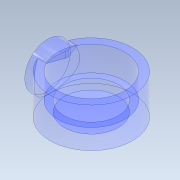
# Autodesk Inventor part: hip_right
Saved by Autodesk Inventor 2020 (Build 240168000, 168)
## iProperties
Created: 2021-03-27
Part Number: hip_right
Material: Generic
Document SubType Name: Modeling
Designer: DELL
Density: 1 g/cm^3
Appearance: Clear - Blue
Author: DELL
Autodesk Inventor part; units mm, degrees
ref_plane "YZ Plane" through (0, 0, 0) normal (1, 0, 0) x (0, 1, 0)
ref_plane "XY Plane" through (0, 0, 0) normal (0, 0, 1) x (1, 0, 0)
ref_plane "UCS1: YZ Plane" through (0, 0, 0) normal (1, 0, 0) x (0, 1, 0)
sketch "Sketch2" plane through (0, 0, 0) normal (1, 0, 0) x (0, 1, 0)
  circle A0 centre (0, 0) radius 26.5
  dimension "d0" = 53
  constraints: 1 centre point, 1 coincident
  measures "d0" diameter of A0
extrude "Extrusion1" add sketch "Sketch2" along normal blind 51
sketch "Sketch3" plane through (0, 0, 0) normal (0, 1, 0) x (-1, 0, 0)
  line L0 (-51, 26.5) -> (-51, -26.5) projected
  circle A0 centre (-51, 0) radius 48
  circle A1 centre (-51, 0) radius 39
  line L1 (-16.6387, 18.4473) -> (-22.6683, 1.8811)
  circle A2 centre (-17.5, 0) radius 5.5
  line L2 (0, 0) -> (-51, 0) construction
  line L3 (0, 26.5) -> (0, -26.5) construction
  line L4 (-16.6387, -18.4473) -> (-22.6683, -1.8811)
  circle A3 centre (-51, 0) radius 31.5
  point P0 (-22.6683, -1.8811)
  point P1 (-20.4946, 7.8532)
  point P2 (-20.4946, -7.8532)
  dimension "d4" = 78
  dimension "d7" = 11
  dimension "d3" = 96
  dimension "d8" = 17.5
  dimension "d9" = 140
  dimension "d15" = 63
  constraints: 6 end point, 2 centre point, 2 coincident, 2 symmetric about line, 1 horizontal, 1 midpoint, 1 point on line, 8 other
  measures "d3" diameter of A0
  measures "d8" distance from line of L3 point (-17.5, 0)
  measures "d9" angle of L4 L1
  measures "d15" diameter of A3
ref_plane "Work Plane1" through (0, -26.5, 0) normal (0, 1, 0) x (-1, 0, 0)
extrude "Extrusion2" add sketch "Sketch3" along normal blind 46 from surface at -26.5 contours A0 | A2 A3 L1 A1 | A2 A3 | A1 L4 A3 A2 | L1 A3 L4 A1 | A3 A2 | A2 L1 A3 | A3 L4 A2 | L1 A2 L4 A3
ref_plane "Work Plane2" through (0, -9.5, 0) normal (0, 1, 0) x (-1, 0, 0)
extrude "Extrusion3" cut sketch "Sketch3" along normal up to surface (29 mm away) from surface at -9.5 contours A2 A3 L1 A1 | A2 A3 | A1 L4 A3 A2 | L1 A3 L4 A1 | A3 A2 | A2 L1 A3 | A3 L4 A2 | L1 A2 L4 A3
extrude "Extrusion4" cut sketch "Sketch3" along normal through all contours L1 A3 L4 A1 | L1 A2 L4 A3
extrude "Extrusion5" cut sketch "Sketch3" against normal blind 12 from surface at -9.5 contours A3 A2 | A2 L1 A3 | A3 L4 A2 | L1 A2 L4 A3 picked at (-20.6688, -0.7652)
body "Solid1"
